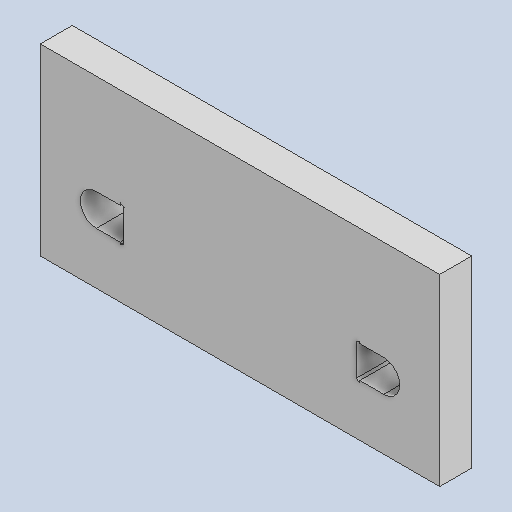
# Autodesk Inventor part: N20Bracklet-Holder
Saved by Autodesk Inventor 2024 (Build 280153000, 153)
## iProperties
Created: 2024-01-13
Part Number: N20Bracklet-Holder
Material: Generic
Document SubType Name: Modeling
Designer: student
Density: 1 g/cm^3
Appearance: Default
Author: student
Autodesk Inventor part; units mm, degrees
ref_plane "YZ Plane" through (0, 0, 0) normal (1, 0, 0) x (0, 1, 0)
ref_plane "XZ Plane" through (0, 0, 0) normal (0, 1, 0) x (-1, 0, 0)
ref_plane "XY Plane" through (0, 0, 0) normal (0, 0, 1) x (1, 0, 0)
sketch "Sketch1" plane through (0, 0, 0) normal (0, 0, 1) x (1, 0, 0)
  line L0 (1.5, -5.75) -> (-1.9843, -5.75) projected
  line L1 (0, 0) -> (1.5, 0) projected
  line L2 (1.5, 0) -> (1.5, 5.75) projected
  line L3 (-16, 5.75) -> (1.5, 5.75) projected
  line L4 (-16, 3.21) -> (-16, 5.75) projected
  line L5 (0, 3.21) -> (-16, 3.21) projected
  line L6 (0, 2.75) -> (0, 3.21) projected
  line L7 (0, 2.75) -> (-1.9843, 2.75) projected
  arc A0 (-1.9843, 2.75) -> (-3.3072, 2.25) centre (-1.9843, 0.75) ccw projected
  arc A1 (-3.3072, 2.25) -> (-3.3072, -5.25) centre (0, -1.5) ccw projected
  arc A2 (-3.3072, -5.25) -> (-1.9843, -5.75) centre (-1.9843, -3.75) ccw projected
  line L8 (1.5, -5.75) -> (-1.9843, -5.75) projected
  line L9 (1.5, -5.75) -> (1.5, -3) projected
  line L10 (1.5, -3) -> (0, -3) projected
  line L11 (0, -3) -> (0, -2.5) projected
  line L12 (0, -2.5) -> (-1.5, -2.5) projected
  arc A3 (-1.5, -0.5) -> (-1.5, -2.5) centre (-1.5, -1.5) ccw projected
  line L13 (-1.5, -0.5) -> (0, -0.5) projected
  line L14 (0, -0.5) -> (0, 0) projected
  line L15 (15, -3) -> (13.5, -3) projected
  line L16 (13.5, -5.75) -> (13.5, -3) projected
  line L17 (13.5, -5.75) -> (16.9843, -5.75) projected
  arc A4 (16.9843, -5.75) -> (18.3072, -5.25) centre (16.9843, -3.75) ccw projected
  arc A5 (18.3072, -5.25) -> (18.3072, 2.25) centre (15, -1.5) ccw projected
  arc A6 (18.3072, 2.25) -> (16.9843, 2.75) centre (16.9843, 0.75) ccw projected
  line L18 (15, 2.75) -> (16.9843, 2.75) projected
  line L19 (15, 2.75) -> (15, 3.21) projected
  line L20 (31, 3.21) -> (15, 3.21) projected
  line L21 (31, 3.21) -> (31, 5.75) projected
  line L22 (13.5, 5.75) -> (31, 5.75) projected
  line L23 (13.5, 0) -> (13.5, 5.75) projected
  line L24 (13.5, 0) -> (15, 0) projected
  line L25 (15, 0) -> (15, -0.5) projected
  line L26 (15, -0.5) -> (16.5, -0.5) projected
  arc A7 (16.5, -2.5) -> (16.5, -0.5) centre (16.5, -1.5) ccw projected
  line L27 (16.5, -2.5) -> (15, -2.5) projected
  line L28 (15, -2.5) -> (15, -3) projected
  line L29 (14.7679, -0.5) -> (15, -0.366) projected
  line L30 (15, 0) -> (15, -0.366) projected
  line L31 (13.5, 0) -> (15, 0) projected
  line L32 (13.5, -3) -> (13.5, 0) projected
  line L33 (15, -3) -> (13.5, -3) projected
  line L34 (15, -2.634) -> (15, -3) projected
  line L35 (15, -2.634) -> (14.7679, -2.5) projected
  line L36 (14.7679, -2.5) -> (14.7679, -0.5) projected
  line L37 (0, -0.366) -> (0.2321, -0.5) projected
  line L38 (0.2321, -0.5) -> (0.2321, -2.5) projected
  line L39 (0.2321, -2.5) -> (0, -2.634) projected
  line L40 (0, -2.634) -> (0, -3) projected
  line L41 (0, -3) -> (1.5, -3) projected
  line L42 (1.5, 0) -> (1.5, -3) projected
  line L43 (1.5, 0) -> (0, 0) projected
  line L44 (0, 0) -> (0, -0.366) projected
  line L45 (20, -1.5) -> (20, -5.75)
  line L46 (13.5, -5.75) -> (20, -5.75)
  line L47 (13.5, -5.75) -> (-1.9843, -5.75)
  line L48 (-5, -1.5) -> (-5, -5.75)
  line L49 (-5, -5.75) -> (-1.9843, -5.75)
  line L50 (20, -5.75) -> (-5, -5.75)
  line L51 (-5, -5.75) -> (-5, 5.75)
  line L52 (-5, 5.75) -> (20, 5.75)
  line L53 (20, 5.75) -> (20, -5.75)
  constraints: 18 end point, 3 perpendicular, 3 point on circle, 2 parallel, 2 point on line, 2 vertical, 1 horizontal, 1 tangent
extrude "Extrusion1" add sketch "Sketch1" along normal blind 2 contours L0 A2 A1 A0 L7 L6 L5 L51 L3 L2 L1 L14 L13 A3 L12 L11 L10 L9 | L9 L42 L2 L52 L23 L32 L16 L47 | L49 L48 A1 A2 | L10 L11 L39 L38 L37 L14 L1 L42 | L16 L15 L28 L27 A7 L26 L25 L24 L23 L22 L53 L20 L19 L18 A6 A5 A4 L17 | L32 L24 L25 L29 L36 L35 L28 L15 | A4 A5 L45 L46 | L51 L5 L6 L7 A0 A1 | A5 A6 L18 L19 L20 L53
body "Solid1"
